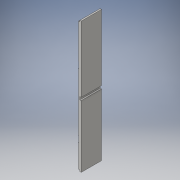
# Autodesk Inventor part: Door Side
Saved by Autodesk Inventor 2016 (Build 200138000, 138)
## iProperties
Created: 2017-10-31
Part Number: Door Side
Material: Generic
Document SubType Name: Modeling
Designer: mathaetaes
Density: 1 g/cm^3
Appearance: Default
Author: mathaetaes
Autodesk Inventor part; units mm, degrees
ref_plane "YZ Plane" through (0, 0, 0) normal (1, 0, 0) x (0, 1, 0)
ref_plane "XZ Plane" through (0, 0, 0) normal (0, 1, 0) x (-1, 0, 0)
ref_plane "XY Plane" through (0, 0, 0) normal (0, 0, 1) x (1, 0, 0)
sketch "Sketch1" plane through (0, 0, 0) normal (0, 1, 0) x (-1, 0, 0)
  line L0 (0, 0) -> (-19.05, 0)
  line L1 (-19.05, 0) -> (-19.05, 133.35)
  line L2 (-19.05, 133.35) -> (0, 133.35)
  line L3 (0, 133.35) -> (0, 0)
  dimension "d0" = 19.05
  dimension "d1" = 133.35
  constraints: 8 end point, 2 parallel, 1 horizontal, 1 perpendicular
  measures "d0" distance of L1.end L2.end
  measures "d1" distance of L0.end L1.end
extrude "Board" add sketch "Sketch1" along normal blind 857.25
sketch "Sketch2" plane through (19.05, 0, 133.35) normal (1, 0, 0) x (0, 0, -1)
  line L0 (0, 425.45) -> (133.35, 425.45)
  line L1 (133.35, 425.45) -> (133.35, 406.4)
  line L2 (133.35, 406.4) -> (0, 406.4)
  line L3 (0, 406.4) -> (0, 425.45)
  line L4 (0, 0) -> (133.35, 0) projected
  line L5 (0, 0) -> (0, 857.25) projected
  line L6 (133.35, 0) -> (133.35, 857.25) projected
  dimension "d4" = 19.05
  dimension "d5" = 406.4
  constraints: 8 end point, 2 collinear, 2 parallel, 1 horizontal, 1 perpendicular
  measures "d4" distance of L0.end L1.end
  measures "d5" distance between parallel lines of L4 L2
extrude "Shelf Notch" cut sketch "Sketch2" against normal blind 9.525 contours L0 L1 L2 L3
sketch "Sketch3" plane through (0, 0, 133.35) normal (0, 0, 1) x (1, 0, 0)
  line L0 (0, 857.25) -> (19.05, 857.25) projected
  line L1 (0, 857.25) -> (9.525, 857.25)
  line L2 (9.525, 857.25) -> (9.525, 847.725)
  line L3 (9.525, 847.725) -> (0, 847.725)
  line L4 (0, 847.725) -> (0, 857.25)
  line L5 (0, 0) -> (9.525, 0)
  line L6 (9.525, 0) -> (9.525, 9.525)
  line L7 (9.525, 9.525) -> (0, 9.525)
  line L8 (0, 9.525) -> (0, 0)
  dimension "d8" = 9.525
  dimension "d9" = 9.525
  dimension "d14" = 9.525
  dimension "d15" = 9.525
  constraints: 16 end point, 4 parallel, 2 horizontal, 2 perpendicular
  measures "d8" distance of L2.end L3.end
  measures "d9" distance of L1.end L2.end
  measures "d14" distance of L7.end L6.end
  measures "d15" distance of L6.end L5.end
extrude "Top and Bottom Dados" cut sketch "Sketch3" against normal blind 133.35
sketch "Sketch5" plane through (0, 9.525, 0) normal (-1, 0, 0) x (0, 0, 1)
  line L0 (122.2375, 609.6) -> (133.35, 609.6)
  line L1 (133.35, 609.6) -> (133.35, 571.5)
  line L2 (133.35, 571.5) -> (122.2375, 571.5)
  line L3 (119.0625, 574.675) -> (119.0625, 606.425)
  line L4 (133.35, 800.1) -> (0, 800.1) projected
  line L5 (133.35, 0) -> (133.35, 838.2) projected
  line L6 (122.2375, 190.5) -> (133.35, 190.5)
  line L7 (133.35, 190.5) -> (133.35, 152.4)
  line L8 (133.35, 152.4) -> (122.2375, 152.4)
  line L9 (119.0625, 155.575) -> (119.0625, 187.325)
  line L10 (0, 0) -> (133.35, 0) projected
  arc A0 (122.2375, 609.6) -> (119.0625, 606.425) centre (122.2375, 606.425) ccw
  arc A1 (119.0625, 574.675) -> (122.2375, 571.5) centre (122.2375, 574.675) ccw
  arc A2 (122.2375, 190.5) -> (119.0625, 187.325) centre (122.2375, 187.325) ccw
  arc A3 (119.0625, 155.575) -> (122.2375, 152.4) centre (122.2375, 155.575) ccw
  point P0 (0, -9.525)
  point P1 (119.0625, 571.5)
  point P2 (119.0625, 152.4)
  dimension "d16" = 14.2875
  dimension "d17" = 38.1
  dimension "d18" = 838.2
  dimension "d19" = 190.5
  dimension "d20" = 38.1
  dimension "d21" = 14.2875
  dimension "d22" = 381
  dimension "d24" = 3.175
  constraints: 16 end point, 8 point on circle, 8 tangent, 4 centre point, 4 parallel, 4 point on line, 3 equal radius, 2 collinear, 2 horizontal, 2 perpendicular
  measures "d16" distance of L1.end point (119.062, 571.5)
  measures "d17" distance of L0.end L1.end
  measures "d18" distance of L5.start L4.start
  measures "d19" distance between parallel lines of L0 L4
  measures "d20" distance of L6.end L7.end
  measures "d21" distance of L7.end point (119.062, 152.4)
  measures "d22" distance between parallel lines of L6 L2
  measures "d24" radius of A0
extrude "Hinge" cut sketch "Sketch5" against normal blind 3.175
equation "\"d12\" = d1"
equation "\"d19\" = 0.25 * d18 - 0.5 * d17"
equation "\"d20\" = d17"
equation "\"d21\" = d16"
equation "\"d22\" = 2 * d19"
body "Solid1"
